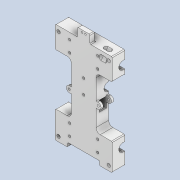
# Autodesk Inventor part: 0008-10-007 Contra suport injectomat
Saved by Autodesk Inventor 2020 (Build 240168000, 168)
## iProperties
Created: 2021-02-26
Part Number: 0008-10-007 Contra suport injectomat
Material: ABS Plastic
Document SubType Name: Modeling
Designer: Iulian Bors
Density: 1.06 g/cm^3
Appearance: Smooth - White
Mass: 601.863 g
Surface Area: 911.871 cm^2
Volume: 567.795 cm^3
Description: Contra suport
Author: Iulian Bors
Subject: 007
Autodesk Inventor part; units mm, degrees
ref_plane "YZ Plane" through (0, 0, 0) normal (1, 0, 0) x (0, 1, 0)
ref_plane "XZ Plane" through (0, 0, 0) normal (0, 1, 0) x (-1, 0, 0)
sketch "Sketch1" plane through (0, 0, 0) normal (0, 0, 1) x (1, 0, 0)
  line L0 (-68, 115) -> (68, 115)
  line L1 (68, 115) -> (68, -115)
  line L2 (68, -115) -> (-68, -115)
  line L3 (-68, -115) -> (-68, 115)
  point P0 (0, 0)
  point P1 (0, 115)
  point P2 (-68, 0)
  dimension "d0" = 230
  dimension "d1" = 136
  constraints: 8 end point, 2 midpoint, 2 parallel, 1 horizontal, 1 horizontal alignment, 1 perpendicular, 1 vertical alignment
  measures "d0" distance of L2.end L0.start
  measures "d1" distance of L1.end L2.end
extrude "Extrusion1" add sketch "Sketch1" along normal blind 30
sketch "Sketch2" plane through (68, -115, 0) normal (1, 0, 0) x (0, 0, -1)
  circle A0 centre (-4.5, 200) radius 9.75
  circle A1 centre (-4.5, 30) radius 9.75
  line L0 (0, 0) -> (-30, 0) projected
  line L1 (0, 0) -> (0, 230) projected
  line L2 (0, 230) -> (-30, 230) projected
  line L3 (-4.5, 209.75) -> (0, 209.75)
  line L4 (-4.5, 190.25) -> (0, 190.25)
  line L5 (-4.5, 39.75) -> (0, 39.75)
  line L6 (-4.5, 20.25) -> (0, 20.25)
  circle A2 centre (-4.5, 30) radius 9.5 projected
  circle A3 centre (-1.5, 135) radius 9.75
  line L7 (-1.5, 144.75) -> (0, 144.75)
  line L8 (0, 125.25) -> (-7.2448, 125.25)
  line L9 (0, 115) -> (-19.3851, 115) construction
  point P0 (-3.9143, 138.0947)
  point P1 (0, 191.3506)
  point P2 (0, 208.6494)
  point P3 (0, 38.6494)
  point P4 (0, 21.3506)
  point P5 (-1.5, 125.25)
  point P6 (0, 125.3661)
  point P7 (0, 144.6339)
  dimension "d4" = 30
  dimension "d6" = 19.5
  dimension "d7" = 30
  dimension "d19" = 4.5
  dimension "d20" = 1.5
  dimension "d28" = 20
  constraints: 14 end point, 9 horizontal, 4 point on circle, 4 tangent, 2 centre point, 1 equal radius, 1 vertical alignment, 12 other
  measures "d4" distance from line of L0 A1.centre
  measures "d6" diameter of A1
  measures "d7" distance from line of A0.centre L2
  measures "d28" distance from line of point (-1.5, 135) L9
extrude "Extrusion2" cut sketch "Sketch2" against normal through all
sketch "Sketch3" plane through (0, 0, 30) normal (0, 0, 1) x (1, 0, 0)
  circle A0 centre (-60, 103.25) radius 4
  circle A1 centre (60, 103.25) radius 4
  circle A2 centre (60, -113.25) radius 4
  circle A3 centre (-60, -113.25) radius 4
  line L0 (68, 115) -> (-68, 115) projected
  line L1 (-68, 115) -> (-68, -115) projected
  line L2 (68, -115) -> (68, 115) projected
  line L3 (-68, -115) -> (68, -115) projected
  point P0 (0, 0)
  dimension "d10" = 11.75
  dimension "d11" = 8
  dimension "d12" = 8
  dimension "d13" = 8
  dimension "d14" = 1.75
  constraints: 4 centre point, 3 equal radius, 2 horizontal alignment, 2 vertical alignment
  measures "d10" distance from line of A0.centre L0
  measures "d11" diameter of A0
  measures "d12" distance from line of A0.centre L1
  measures "d13" distance from line of L2 A1.centre
  measures "d14" distance from line of L3 A2.centre
extrude "Extrusion3" cut sketch "Sketch3" against normal through all contours A0 | A1 | A2 L3 | L3 A2 | L3 A3 | A3 L3
sketch "Sketch5" plane through (0, 0, 30) normal (0, 0, 1) x (1, 0, 0)
  line L0 (-68, 75.25) -> (68, 75.25) projected
  line L1 (68, -75.25) -> (-68, -75.25) projected
  line L2 (-68, 62.75) -> (-29.5, 62.75)
  line L3 (-29.5, 62.75) -> (-29.5, -60.25)
  line L4 (-29.5, -60.25) -> (-68, -60.25)
  line L5 (-68, -60.25) -> (-68, 62.75)
  line L6 (-14.5, 30.7059) -> (14.5, 30.7059) construction
  line L7 (-68, 115) -> (-68, -115) construction
  point P0 (0, 0)
  point P1 (0, 30.7059)
  dimension "d21" = 29
  dimension "d22" = 15
  dimension "d23" = 12.5
  dimension "d24" = 15
  constraints: 10 end point, 2 horizontal, 2 parallel, 1 collinear, 1 midpoint, 1 perpendicular, 1 vertical alignment
  measures "d21" distance of L6.start L6.end
  measures "d22" distance from line of L6.start L3
  measures "d23" distance between parallel lines of L2 L0
  measures "d24" distance between parallel lines of L1 L4
extrude "Extrusion4" cut sketch "Sketch5" against normal blind 47
mirror "Mirror1" about plane through (0, 0, 0) normal (1, 0, 0) of "Extrusion4"
sketch "Sketch6" plane through (-29.5, 20, 1.5) normal (-1, 0, 0) x (0, 0, 1)
  line L0 (-1.5, -80.25) -> (-1.5, -9.75) projected
  line L1 (28.5, -80.25) -> (28.5, 42.75) projected
  line L2 (-1.5, -15.5) -> (28.5, -15.5)
  line L3 (28.5, -15.5) -> (28.5, -30.5)
  line L4 (28.5, -30.5) -> (-1.5, -30.5)
  line L5 (-1.5, -30.5) -> (-1.5, -15.5)
  line L6 (-1.5, -23) -> (28.5, -23) construction
  line L7 (-1.5, -15.5) -> (3.5, -15.5)
  line L8 (3.5, -15.5) -> (3.5, -30.5)
  line L9 (3.5, -30.5) -> (-1.5, -30.5)
  line L10 (-1.5, -30.5) -> (-1.5, -15.5)
  line L11 (28.5, -15.5) -> (23.5, -15.5)
  line L12 (23.5, -15.5) -> (23.5, -30.5)
  line L13 (23.5, -30.5) -> (28.5, -30.5)
  line L14 (28.5, -30.5) -> (28.5, -15.5)
  point P0 (-1.5, -20)
  point P1 (-1.5, -70.25)
  point P2 (28.5, -70.25)
  point P3 (28.5, 30.25)
  point P4 (-1.5, -30.5)
  point P5 (28.5, -15.5)
  point P6 (23.5, -15.5)
  point P7 (3.5, -15.5)
  dimension "d29" = 15
  dimension "d31" = 3
  dimension "d38" = 5
  dimension "d39" = 5
  constraints: 26 end point, 6 parallel, 4 point on line, 3 horizontal, 3 perpendicular, 2 midpoint
  measures "d29" distance between parallel lines of L4 L2
  measures "d31" distance from line of L6 point (-1.5, -20)
  measures "d38" distance between parallel lines of L3 L12
  measures "d39" distance between parallel lines of L5 L8
extrude "Extrusion5" add sketch "Sketch6" along normal blind 12 contours L0 L2 L8 L4 | L12 L2 L1 L4
sketch "Sketch8" plane through (0, 0, 30) normal (0, 0, 1) x (1, 0, 0)
  circle A0 centre (-34.5, -3) radius 2.5
  line L0 (-29.5, 62.75) -> (-29.5, 4.5) projected
  line L1 (-41.5, -10.5) -> (-41.5, 4.5) projected
  point P0 (0, 0)
  point P1 (-29.5, 50.25)
  point P2 (-41.5, -3)
  dimension "d40" = 5
  dimension "d41" = 5
  constraints: 1 centre point, 1 horizontal alignment, 1 midpoint
  measures "d40" diameter of A0
  measures "d41" distance from line of L0 A0.centre
extrude "Extrusion6" cut sketch "Sketch8" against normal through all
fillet "Fillet2" radius 7.5 4 edges at (-41.5, 4.5, 27.5) (-41.5, -10.5, 27.5) (-41.5, 4.5, 2.5) (-41.5, -10.5, 2.5)
mirror "Mirror2" about plane through (0, 0, 0) normal (1, 0, 0) of "Extrusion5", "Extrusion6", "Fillet2"
sketch "Sketch9" plane through (0, 0, 30) normal (0, 0, 1) x (1, 0, 0)
  circle A0 centre (-60, 103.25) radius 4 projected
  line L0 (68, 115) -> (-68, 115) projected
  line L1 (68, 94.75) -> (-68, 94.75) projected
  line L2 (-68, 75.25) -> (68, 75.25) projected
  line L3 (-68, 62.75) -> (-29.5, 62.75) projected
  line L4 (-68, 115) -> (-68, -115) projected
  point P0 (0, 0)
  point P1 (-33.5, 100)
  point P2 (-33.5, 72.75)
  point P3 (-58, 60.25)
  point P4 (-39.5, 60.25)
  point P5 (-68, 70.25)
  point P6 (-29.5, 62.75)
  dimension "d59" = 15
  dimension "d60" = 10
  dimension "d70" = 34.5
  constraints: 1 vertical alignment, 1 other
  measures "d59" distance from line of L0 point (-33.5, 100)
  measures "d70" distance from line of point (-33.5, 100) L4
hole "Hole1" at (-33.5, 100, 30) at (-33.5, 72.75, 30) direction (0, 0, -1) diameter 5.5 end through all
mirror "Mirror3" about plane through (0, 0, 0) normal (1, 0, 0) of "Hole1"
mirror "Mirror4" about plane through (0, 0, 0) normal (0, 1, 0) of "Hole1", "Mirror3"
sketch "Sketch10" plane through (0, 0, 0) normal (0, 0, -1) x (-1, 0, 0)
  line L0 (-29.5, 29.75) -> (29.5, 29.75) projected
  line L1 (29.5, 10.25) -> (-29.5, 10.25) projected
  point P0 (0, 0)
  point P1 (0, 37.25)
  point P2 (0, 2.75)
  dimension "d61" = 7.5
  dimension "d62" = 7.5
  constraints: 2 vertical alignment
  measures "d61" distance from line of L0 point (0, 37.25)
  measures "d62" distance from line of L1 point (0, 2.75)
hole "Hole2" at (0, 37.25, 0) at (0, 2.75, 0) direction (0, 0, 1) diameter 5.5 end through all
sketch "Sketch11" plane through (-29.5, 20, 1.5) normal (-1, 0, 0) x (0, 0, 1)
  line L0 (3.5, -17.5) -> (21, -17.5)
  line L1 (21, -17.5) -> (21, -42.5)
  line L2 (21, -42.5) -> (3.5, -42.5)
  line L3 (3.5, -42.5) -> (3.5, -17.5)
  line L4 (-1.5, 95) -> (28.5, 95) projected
  line L5 (3.5, -15.5) -> (-1.5, -15.5) projected
  line L6 (23.5, -30.5) -> (28.5, -30.5) projected
  line L7 (23.5, -30.5) -> (23.5, -15.5) projected
  line L8 (3.5, -15.5) -> (3.5, -30.5) projected
  point P0 (-1.5, -20)
  point P1 (13.5, 95)
  dimension "d78" = 2.5
  dimension "d79" = 0
  dimension "d80" = 25
  dimension "d81" = 112.5
  constraints: 8 end point, 2 parallel, 1 horizontal, 1 midpoint, 1 perpendicular
  measures "d78" distance between parallel lines of L7 L1
  measures "d79" distance between parallel lines of L3 L8
  measures "d80" distance of L0.end L1.end
  measures "d81" distance between parallel lines of L0 L4
extrude "Extrusion7" cut sketch "Sketch11" against normal through all
sketch "Sketch13" plane through (0, 0, 30) normal (0, 0, 1) x (1, 0, 0)
  line L0 (-15, 135) -> (15, 135)
  line L1 (15, 135) -> (15, 115)
  line L2 (15, 115) -> (-15, 115)
  line L3 (-15, 115) -> (-15, 135)
  line L4 (68, 115) -> (-68, 115) projected
  point P0 (0, 0)
  point P1 (0, 135)
  point P2 (0, 115)
  point P3 (0, 115)
  dimension "d86" = 20
  dimension "d87" = 30
  constraints: 8 end point, 3 midpoint, 2 parallel, 1 coincident, 1 collinear, 1 horizontal, 1 perpendicular, 1 vertical alignment
  measures "d86" distance of L2.end L0.start
  measures "d87" distance of L0.start L0.end
extrude "Extrusion9" add sketch "Sketch13" against normal blind 10
sketch "Sketch14" plane through (0, 0, 30) normal (0, 0, 1) x (1, 0, 0)
  line L0 (-15, 135) -> (-15, 115) projected
  line L1 (15, 115) -> (15, 135) projected
  line L2 (0, 126.2256) -> (0, 115) construction
  line L3 (68, 115) -> (-68, 115) construction
  line L4 (15, 135) -> (-15, 135) construction
  line L5 (-15, 135) -> (15, 135) projected
  point P0 (0, 0)
  point P1 (-4, 130)
  point P2 (4, 130)
  point P3 (-15, 125)
  point P4 (15, 125)
  point P5 (0, 120.6128)
  point P6 (0, 135)
  dimension "d90" = 8
  dimension "d91" = 4
  dimension "d127" = 5
  constraints: 5 midpoint, 2 end point, 1 horizontal alignment, 1 vertical, 1 vertical alignment
  measures "d90" distance of point (4, 130) point (-4, 130)
  measures "d91" distance from line of L2 point (-4, 130)
  measures "d127" distance from line of L5 point (-4, 130)
hole "Hole3" at (-4, 130, 30) at (4, 130, 30) direction (0, 0, -1) diameter 4 end through all
fillet "Fillet3" radius 2 5 edges at (15, 115, 25) (15, 135, 25) (-15, 135, 25) (-15, 115, 25) (0, 115, 20)
sketch "Sketch15" plane through (0, 0, 30) normal (0, 0, 1) x (1, 0, 0)
  line L0 (-68, -115) -> (-38, -115)
  line L1 (-38, -115) -> (-38, -125)
  line L2 (-38, -125) -> (-68, -125)
  line L3 (-68, -125) -> (-68, -115)
  line L4 (38, -115) -> (68, -115)
  line L5 (68, -115) -> (68, -125)
  line L6 (68, -125) -> (38, -125)
  line L7 (38, -125) -> (38, -115)
  line L8 (-56.4031, -115) -> (56.4031, -115) projected
  line L9 (68, -115) -> (68, 115) projected
  line L10 (-68, -60.25) -> (-68, -115) projected
  circle A0 centre (-60, -113.25) radius 4
  circle A1 centre (60, -113.25) radius 4
  arc A2 (-56.4031, -115) -> (-63.5969, -115) centre (-60, -113.25) ccw projected
  arc A3 (63.5969, -115) -> (56.4031, -115) centre (60, -113.25) ccw projected
  point P0 (0, 0)
  point P1 (68, -70.25)
  point P2 (-68, -70.25)
  dimension "d100" = 30
  dimension "d101" = 10
  constraints: 16 end point, 4 collinear, 4 parallel, 2 centre point, 2 concentric, 2 equal length, 2 equal radius, 2 horizontal, 2 perpendicular
  measures "d100" distance of L1.end L2.end
  measures "d101" distance of L2.end L0.start
extrude "Extrusion10" add sketch "Sketch15" against normal up to surface (30 mm away) contours L4 A1 L5 L6 L7 | L0 A0 L1 L2 L3
fillet "Fillet4" radius 2 10 edges at (68, 115, 15) (68, 62.75, 15) (-68, 115, 15) (-68, 62.75, 15) (-68, -60.25, 15) (68, -60.25, 15) (-38, -115, 15) (-38, -125, 15) (38, -115, 15) (38, -125, 15)
fillet "Fillet5" radius 10 4 edges at (-29.5, 62.75, 15) (-29.5, -60.25, 15) (29.5, 62.75, 15) (29.5, -60.25, 15)
sketch "Sketch17" plane through (66, 62.75, 0) normal (0, -1, 0) x (1, 0, 0)
  circle A0 centre (-1.1275, 12.7125) radius 1.7875 projected
  point P0 (-66, 0)
hole "Hole5" at (64.8725, 62.75, 12.7125) direction (0, 1, 0) diameter 2.459 depth 8.8 tip angle 118 thread size "M3x0.5" class "6H" standard "ISO Metric profile"
ref_plane "Work Plane1" through (68, 115, 30) normal (0, -0.7831, 0.6219) x (-1, 0, 0)
sketch "Sketch19" plane through (68, 115, 30) normal (0, -0.7831, 0.6219) x (-1, 0, 0)
  line L0 (16.5, 9) -> (26.5, 9) construction
  line L1 (16.5, 5) -> (26.5, 5)
  line L2 (26.5, 13) -> (16.5, 13)
  arc A0 (16.5, 13) -> (16.5, 5) centre (16.5, 9) ccw
  arc A1 (26.5, 5) -> (26.5, 13) centre (26.5, 9) ccw
  line L3 (0, 1.2438) -> (0, 24.7371) projected
  line L4 (2, 0) -> (51, 0) projected
  point P0 (68, 95.0098)
  point P1 (21.5, 9)
  dimension "d120" = 10
  dimension "d121" = 8
  dimension "d122" = 21.5
  dimension "d124" = 5
  constraints: 8 end point, 4 point on circle, 4 tangent, 2 centre point, 1 horizontal, 1 midpoint, 1 parallel
  measures "d120" distance of L0.start L0.end
  measures "d121" distance between parallel lines of L2 L1
  measures "d122" distance from line of point (21.5, 9) L3
  measures "d124" distance between parallel lines of L1 L4
extrude "Extrusion11" cut sketch "Sketch19" along normal through all both and the other way through all
equation "\"d13\" = d12"
equation "\"d91\" = 0.5 * d90"
body "Solid1"
